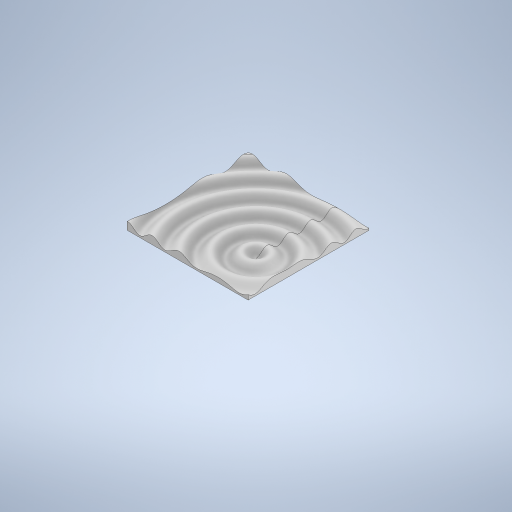
# Autodesk Inventor part: wave_plate
Saved by Autodesk Inventor 2024.3 (Build 283343000, 343)
## iProperties
Created: 2024-06-19
Part Number: wave_plate
Material: Generic
Document SubType Name: Modeling
Designer: hugodrak
Density: 1 g/cm^3
Appearance: Default
Author: hugodrak
## iProperties of the stored document wave_plate_3DPrint.ipt
Created: 2024-06-19
Part Number: wave_plate_3DPrint
Material: Generic
Document SubType Name: Modeling
Designer: hugodrak
Density: 1 g/cm^3
Appearance: Default
Author: hugodrak
Autodesk Inventor part; units mm, degrees
ref_plane "YZ Plane" through (0, 0, 0) normal (1, 0, 0) x (0, 1, 0)
ref_plane "XZ Plane" through (0, 0, 0) normal (0, 1, 0) x (-1, 0, 0)
sketch "Sketch1" plane through (0, 0, 0) normal (0, 1, 0) x (-1, 0, 0)
  line L0 (0, 0) -> (200, 0)
  line L1 (200, 0) -> (200, -200)
  line L2 (200, -200) -> (0, -200)
  line L3 (0, -200) -> (0, 0)
  dimension "d0" = 200
  dimension "d1" = 200
  constraints: 8 end point, 2 parallel, 1 horizontal, 1 perpendicular
  measures "d0" distance of L1.end L2.end
  measures "d1" distance of L0.end L1.end
extrude "Extrusion1" add sketch "Sketch1" along normal blind 20
sketch "Sketch2" plane through (0, 0, 0) normal (1, 0, 0) x (0, 0, -1)
  line L0 (200, 0) -> (200, 20) projected
  point P0 (200, 10)
  point P1 (217.3153, 12.9818)
  constraints: 1 midpoint, 1 vertical alignment, 8 other
ref_plane "Work Plane1" through (-50, 0, 0) normal (1, 0, 0) x (0, 0, -1)
sketch "Sketch3" plane through (-50, 0, 0) normal (1, 0, 0) x (0, 0, -1)
  spline S0 degree 3 poles (0, 15) (1.8689, 16.6309) (3.7379, 18.2381) (5.6068, 19.1485) (7.3428, 19.9942) (9.0788, 20.2231) (10.8148, 19.7513) (12.724, 19.2323) (14.6332, 17.8708) (16.5424, 16.2583) (18.5974, 14.5227) (20.6524, 12.5602) (22.7074, 11.3388) (24.4306, 10.3147) (26.1537, 9.8292) (27.8769, 10.0584) (29.7075, 10.302) (31.5382, 11.3517) (33.3688, 12.7837) (35.7685, 14.6609) (38.1682, 17.1141) (40.568, 18.5772) (42.289, 19.6265) (44.0099, 20.1504) (45.7309, 19.9594) (47.553, 19.7571) (49.375, 18.7531) (51.1971, 17.3496) (53.7888, 15.3532) (56.3805, 12.6476) (58.9722, 11.1854) (60.6897, 10.2164) (62.4072, 9.8037) (64.1247, 10.096) (65.9683, 10.4098) (67.812, 11.5347) (69.6556, 13.0107) (72.055, 14.9318) (74.4544, 17.3606) (76.8538, 18.747) (78.5711, 19.7392) (80.2883, 20.1848) (82.0055, 19.9232) (83.8205, 19.6467) (85.6355, 18.5818) (87.4505, 17.1522) (89.6645, 15.4082) (91.8786, 13.1844) (94.0926, 11.7246) (95.8299, 10.5791) (97.5672, 9.9265) (99.3045, 10.0071) (101.1095, 10.0907) (102.9144, 10.9671) (104.7194, 12.291) (106.8275, 13.8373) (108.9357, 15.947) (111.0439, 17.5331) (112.8166, 18.8668) (114.5892, 19.7971) (116.3618, 19.969) (118.1072, 20.1383) (119.8525, 19.5699) (121.5979, 18.4746) (123.9901, 16.9735) (126.3823, 14.5199) (128.7745, 12.6724) (130.5581, 11.2948) (132.3417, 10.2949) (134.1253, 10.0582) (135.8592, 9.828) (137.5931, 10.3222) (139.327, 11.3594) (142.2668, 13.1178) (145.2065, 16.3882) (148.1462, 18.3106) (149.8745, 19.4409) (151.6027, 20.0787) (153.331, 19.9917) (155.1172, 19.9017) (156.9034, 19.0365) (158.6896, 17.7308) (161.295, 15.8262) (163.9005, 13.0669) (166.5059, 11.4608) (168.2279, 10.3993) (169.95, 9.8585) (171.672, 10.0343) (173.4907, 10.2201) (175.3095, 11.2056) (177.1282, 12.5975) (179.6881, 14.5566) (182.2479, 17.2277) (184.8077, 18.7202) (186.5254, 19.7218) (188.2432, 20.1801) (189.9609, 19.9298) (191.7729, 19.6659) (193.5848, 18.6152) (195.3968, 17.1944) (197.576, 15.4856) (199.7552, 13.3008) (201.9345, 11.8301) (203.672, 10.6574) (205.4096, 9.9627) (207.1472, 10.0016) (208.9324, 10.0417) (210.7176, 10.8576) (212.5028, 12.1342) (214.7836, 13.7651) (217.0643, 16.0954) (219.3451, 17.7561) (221.0796, 19.0191) (222.8142, 19.8654) (224.5487, 19.9845) (226.2947, 20.1044) (228.0407, 19.4842) (229.7867, 18.3543) (232.7123, 16.461) (235.6378, 13.2108) (238.5634, 11.4256) (240.2835, 10.3759) (242.0037, 9.8507) (243.7238, 10.0398) (245.607, 10.2469) (247.4902, 11.3136) (249.3734, 12.7873) (251.4828, 14.4381) (253.5923, 16.5404) (255.7017, 18.0103) (257.4538, 19.2311) (259.2059, 19.9886) (260.958, 19.9999) (262.7226, 20.0112) (264.4872, 19.2645) (266.2518, 18.0425) (269.0642, 16.095) (271.8765, 13.0271) (274.6889, 11.3499) (276.4091, 10.3239) (278.1293, 9.8331) (279.8495, 10.0549) (281.6724, 10.2899) (283.4953, 11.3245) (285.3182, 12.7442) (287.7652, 14.6499) (290.2121, 17.1649) (292.6591, 18.6323) (294.3782, 19.6633) (296.0972, 20.1623) (297.8163, 19.9493) (298.5442, 19.8591) (299.2721, 19.6477) (300, 19.3301) knots 0 0 0 0 5.606787 5.606787 5.606787 10.814849 10.814849 10.814849 16.542409 16.542409 16.542409 22.707383 22.707383 22.707383 27.876893 27.876893 27.876893 33.368784 33.368784 33.368784 40.567973 40.567973 40.567973 45.730919 45.730919 45.730919 51.197108 51.197108 51.197108 58.972198 58.972198 58.972198 64.124723 64.124723 64.124723 69.65558 69.65558 69.65558 76.853843 76.853843 76.853843 82.005531 82.005531 82.005531 87.450451 87.450451 87.450451 94.092625 94.092625 94.092625 99.30455 99.30455 99.30455 104.719356 104.719356 104.719356 111.043934 111.043934 111.043934 116.361802 116.361802 116.361802 121.597891 121.597891 121.597891 128.774452 128.774452 128.774452 134.12525 134.12525 134.12525 139.327046 139.327046 139.327046 148.146243 148.146243 148.146243 153.330998 153.330998 153.330998 158.689604 158.689604 158.689604 166.505919 166.505919 166.505919 171.671968 171.671968 171.671968 177.128225 177.128225 177.128225 184.807711 184.807711 184.807711 189.960927 189.960927 189.960927 195.396757 195.396757 195.396757 201.93446 201.93446 201.93446 207.147197 207.147197 207.147197 212.502845 212.502845 212.502845 219.345055 219.345055 219.345055 224.548736 224.548736 224.548736 229.786712 229.786712 229.786712 238.563373 238.563373 238.563373 243.723789 243.723789 243.723789 249.373385 249.373385 249.373385 255.701712 255.701712 255.701712 260.95795 260.95795 260.95795 266.251824 266.251824 266.251824 274.688868 274.688868 274.688868 279.849502 279.849502 279.849502 285.318216 285.318216 285.318216 292.659108 292.659108 292.659108 297.816305 297.816305 297.816305 300 300 300 300 projected
  line L0 (200, 0) -> (0, 0) projected
  line L1 (0, 0) -> (0, 20) projected
  line L2 (200, 20) -> (0, 20) projected
  line L3 (200, 0) -> (200, 20) projected
  line L4 (63.0629, 10.0038) -> (63.0629, 0)
  line L5 (63.0629, 0) -> (63.0629, 20)
  line L6 (200, 20) -> (301.5664, 20)
  line L7 (300, 19.3301) -> (301.5664, 20)
  point P0 (260.9975, 20)
  constraints: 8 end point, 3 point on line, 1 horizontal, 1 perpendicular, 1 other
revolve "Revolution1" cut sketch "Sketch3" angle 360 about axis through (-50, 0, -63.0629) along (0, 1, 0) picked at (100.8114, 15.9988) contours L6 L7 S0 | L6 S0 | L5 L2 S0 | L2 S0 | L2 L3 S0 | L3 L6 S0
sketch "Sketch4" plane through (0, 0, 0) normal (0, -1, 0) x (1, 0, 0)
  line L0 (0, -200) -> (-200, -200) projected
  line L1 (0, 0) -> (0, -200) projected
  line L2 (-200, 0) -> (0, 0) projected
  line L3 (-200, -200) -> (-200, 0) projected
extrude "Extrusion2" cut sketch "Sketch4" against normal blind 7
body "Solid1"
